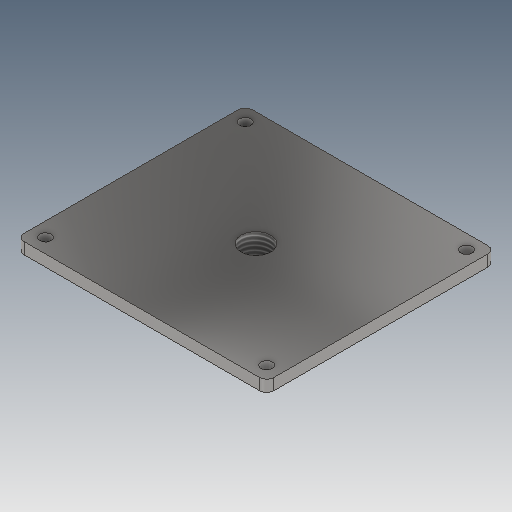
# Autodesk Inventor part: 盖板
Saved by Autodesk Inventor 2025 (Build 290162000, 162)
## iProperties
Created: 2025-03-16
Part Number: 盖板
Material: 聚碳酸酯，透明
Document SubType Name: Modeling
Designer: ASUS
Density: 1.2 g/cm^3
Appearance: 钢 - 抛光
Author: ASUS
Autodesk Inventor part; units mm, degrees
ref_plane "YZ Plane" through (0, 0, 0) normal (1, 0, 0) x (0, 1, 0)
ref_plane "XZ Plane" through (0, 0, 0) normal (0, 1, 0) x (-1, 0, 0)
ref_plane "XY Plane" through (0, 0, 0) normal (0, 0, 1) x (1, 0, 0)
sketch "草图1" plane through (0, 0, 0) normal (0, 1, 0) x (-1, 0, 0)
  line L0 (-5, 0) -> (-170, 0)
  line L1 (-175, 5) -> (-175, 155)
  line L2 (-170, 160) -> (-5, 160)
  line L3 (0, 155) -> (0, 5)
  line L4 (22.306, 80) -> (-199.7113, 80)
  line L5 (-87.5, 206.246) -> (-87.5, -79.95)
  circle A0 centre (-10, 150) radius 4
  circle A1 centre (-10, 10) radius 4
  circle A2 centre (-165, 150) radius 4
  circle A3 centre (-165, 10) radius 4
  arc A4 (0, 155) -> (-5, 160) centre (-5, 155) ccw
  arc A5 (-5, 0) -> (0, 5) centre (-5, 5) ccw
  arc A6 (-175, 5) -> (-170, 0) centre (-170, 5) ccw
  arc A7 (-170, 160) -> (-175, 155) centre (-170, 155) ccw
  point P0 (0, 0)
  point P1 (-175, 0)
  point P2 (0, 160)
  point P3 (-87.5, 160)
  point P4 (0, 80)
  point P5 (-87.5, 80)
  point P6 (-87.5, 0)
  point P7 (-87.5, 80)
  dimension "d0" = 160
  dimension "d1" = 175
  dimension "d2" = 8
  dimension "d6" = 140
  dimension "d9" = 155
  dimension "d12" = 5
  constraints: 12 end point, 10 point on line, 8 centre point, 8 point on circle, 8 tangent, 3 equal radius, 3 horizontal, 2 midpoint, 2 parallel, 2 vertical, 1 perpendicular, 8 other
  measures "d0" distance of point (0, 160) point (0, 0)
  measures "d1" distance of point (0, 0) point (-175, 0)
  measures "d2" diameter of A0
  measures "d6" distance of A0.centre A1.centre
  measures "d9" distance of A0.centre A2.centre
  measures "d12" radius of A4
extrude "拉伸1" add sketch "草图1" along normal blind 8
sketch "草图2" plane through (0, 0, 0) normal (0, -1, 0) x (1, 0, 0)
  line L0 (150, 140) -> (25, 140)
  line L1 (20, 135) -> (20, 25)
  line L2 (25, 20) -> (150, 20)
  line L3 (155, 25) -> (155, 135)
  arc A0 (155, 135) -> (150, 140) centre (150, 135) ccw
  arc A1 (150, 20) -> (155, 25) centre (150, 25) ccw
  arc A2 (20, 25) -> (25, 20) centre (25, 25) ccw
  arc A3 (25, 140) -> (20, 135) centre (25, 135) ccw
  line L4 (87.5, 206.246) -> (87.5, -79.95) projected
  line L5 (-22.306, 80) -> (199.7113, 80) projected
  point P0 (0, 0)
  point P1 (87.5, 140)
  point P2 (155, 80)
  dimension "d15" = 5
  dimension "d16" = 120
  dimension "d17" = 135
  constraints: 8 end point, 8 point on circle, 8 tangent, 4 centre point, 3 equal radius, 2 midpoint, 2 parallel, 2 point on line, 1 horizontal, 1 perpendicular
  measures "d15" radius of A0
  measures "d16" distance between parallel lines of L2 L0
  measures "d17" distance between parallel lines of L1 L3
extrude "拉伸2" cut sketch "草图2" against normal blind 1.5
fillet "圆角1" radius 2 8 edges at (153.5355, 1.5, 138.5355) (155, 1.5, 80) (153.5355, 1.5, 21.4645) (87.5, 1.5, 20) (21.4645, 1.5, 21.4645) (20, 1.5, 80) (21.4645, 1.5, 138.5355) (87.5, 1.5, 140)
sketch "草图3" plane through (0, 1.5, 0) normal (0, -1, 0) x (1, 0, 0)
  line L0 (71.5, 96) -> (103.5, 96)
  line L1 (103.5, 96) -> (103.5, 64)
  line L2 (103.5, 64) -> (71.5, 64)
  line L3 (71.5, 64) -> (71.5, 96)
  line L4 (-22.306, 80) -> (199.7113, 80) projected
  line L5 (87.5, 206.246) -> (87.5, -79.95) projected
  point P0 (0, 0)
  point P1 (71.5, 80)
  point P2 (87.5, 96)
  dimension "d28" = 32
  constraints: 8 end point, 2 midpoint, 2 parallel, 2 perpendicular, 2 point on line, 1 horizontal
  measures "d28" distance of L2.end L0.start
extrude "拉伸3" add sketch "草图3" along normal blind 8.5
fillet "圆角2" radius 2 12 edges at (87.5, -7, 96) (103.5, -7, 80) (87.5, -7, 64) (71.5, -7, 80) (87.5, 1.5, 96) (71.5, 1.5, 80) (103.5, 1.5, 80) (87.5, 1.5, 64) (71.5, -2.75, 96) (71.5, -2.75, 64) (103.5, -2.75, 64) (103.5, -2.75, 96)
sketch "草图4" plane through (0, -7, 0) normal (0, -1, 0) x (1, 0, 0)
  line L0 (-22.306, 80) -> (199.7113, 80) projected
  line L1 (87.5, 206.246) -> (87.5, -79.95) projected
  point P0 (0, 0)
  point P1 (87.5, 80)
  constraints: 2 point on line
hole "孔2" at (87.5, -7, 80) direction (0, 1, 0) diameter 20.752 end through all thread size "M24x3" designation "M24" class "6H" standard "GB Metric profile"
equation "\"d0\" = A1"
equation "\"d1\" = B1"
equation "\"d2\" = d4"
equation "\"d6\" = A2"
equation "\"d9\" = B2"
equation "\"d12\" = R"
equation "\"d13\" = h_"
equation "\"d15\" = R"
equation "\"d16\" = A_"
equation "\"d17\" = B"
equation "\"d4\" = 8"
equation "\"A2\" = 140"
equation "\"B2\" = 155"
equation "\"R\" = 5"
equation "\"h_\" = 8"
equation "\"A_\" = 120"
equation "\"B\" = 135"
equation "\"A1\" = 160"
equation "\"B1\" = 175"
